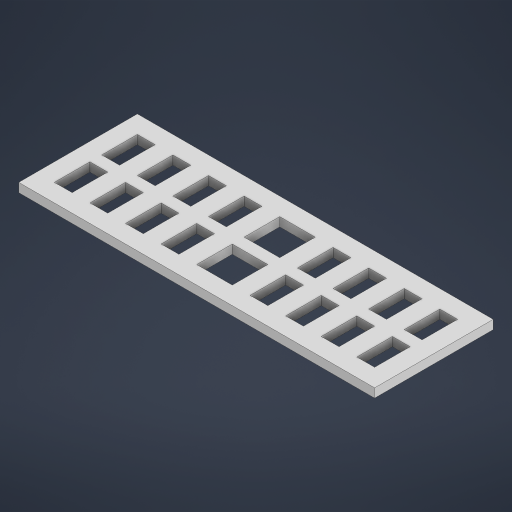
# Autodesk Inventor part: JARING
Saved by Autodesk Inventor 2024 (Build 280153000, 153)
## iProperties
Created: 2025-06-23
Part Number: JARING
Material: Generic
Document SubType Name: Modeling
Designer: ASUS
Density: 1 g/cm^3
Appearance: Default
Author: ASUS
Autodesk Inventor part; units mm, degrees
ref_plane "YZ Plane" through (0, 0, 0) normal (1, 0, 0) x (0, 1, 0)
ref_plane "XZ Plane" through (0, 0, 0) normal (0, 1, 0) x (-1, 0, 0)
ref_plane "XY Plane" through (0, 0, 0) normal (0, 0, 1) x (1, 0, 0)
sketch "Sketch1" plane through (0, 0, 0) normal (0, 1, 0) x (-1, 0, 0)
  line L0 (30, -10) -> (-30, -10)
  line L1 (-30, -10) -> (-30, 10)
  line L2 (-30, 10) -> (30, 10)
  line L3 (30, 10) -> (30, -10)
  line L4 (24, -7) -> (27, -7)
  line L5 (27, -1) -> (24, -1)
  line L6 (27, 1) -> (24, 1)
  line L7 (27, 7) -> (24, 7)
  line L8 (27, -7) -> (27, -1)
  line L9 (27, 1) -> (27, 7)
  line L10 (24, -7) -> (24, -1)
  line L11 (24, 1) -> (24, 7)
  line L12 (-27, -7) -> (-24, -7)
  line L13 (-24, -1) -> (-27, -1)
  line L14 (-24, 1) -> (-27, 1)
  line L15 (-24, 7) -> (-27, 7)
  line L16 (18, -7) -> (21, -7)
  line L17 (21, -1) -> (18, -1)
  line L18 (21, 1) -> (18, 1)
  line L19 (21, 7) -> (18, 7)
  line L20 (-21, -7) -> (-18, -7)
  line L21 (-18, -1) -> (-21, -1)
  line L22 (-18, 1) -> (-21, 1)
  line L23 (-18, 7) -> (-21, 7)
  line L24 (12, -7) -> (15, -7)
  line L25 (15, -1) -> (12, -1)
  line L26 (15, 1) -> (12, 1)
  line L27 (15, 7) -> (12, 7)
  line L28 (-15, -7) -> (-12, -7)
  line L29 (-12, -1) -> (-15, -1)
  line L30 (-12, 1) -> (-15, 1)
  line L31 (-12, 7) -> (-15, 7)
  line L32 (6, -7) -> (9, -7)
  line L33 (9, -1) -> (6, -1)
  line L34 (9, 1) -> (6, 1)
  line L35 (9, 7) -> (6, 7)
  line L36 (-9, -7) -> (-6, -7)
  line L37 (-3, -7) -> (3, -7)
  line L38 (3, -1) -> (-3, -1)
  line L39 (-6, -1) -> (-9, -1)
  line L40 (3, 1) -> (-3, 1)
  line L41 (-6, 1) -> (-9, 1)
  line L42 (3, 7) -> (-3, 7)
  line L43 (-6, 7) -> (-9, 7)
  line L44 (21, -7) -> (21, -1)
  line L45 (21, 1) -> (21, 7)
  line L46 (18, -7) -> (18, -1)
  line L47 (18, 1) -> (18, 7)
  line L48 (15, -7) -> (15, -1)
  line L49 (15, 1) -> (15, 7)
  line L50 (12, -7) -> (12, -1)
  line L51 (12, 1) -> (12, 7)
  line L52 (9, -7) -> (9, -1)
  line L53 (9, 1) -> (9, 7)
  line L54 (6, -7) -> (6, -1)
  line L55 (6, 1) -> (6, 7)
  line L56 (3, -7) -> (3, -1)
  line L57 (3, 1) -> (3, 7)
  line L58 (-3, -7) -> (-3, -1)
  line L59 (-3, 1) -> (-3, 7)
  line L60 (-6, -7) -> (-6, -1)
  line L61 (-6, 1) -> (-6, 7)
  line L62 (-9, -7) -> (-9, -1)
  line L63 (-9, 1) -> (-9, 7)
  line L64 (-12, -7) -> (-12, -1)
  line L65 (-12, 1) -> (-12, 7)
  line L66 (-15, -7) -> (-15, -1)
  line L67 (-15, 1) -> (-15, 7)
  line L68 (-18, -7) -> (-18, -1)
  line L69 (-18, 1) -> (-18, 7)
  line L70 (-21, -7) -> (-21, -1)
  line L71 (-21, 1) -> (-21, 7)
  line L72 (-24, -7) -> (-24, -1)
  line L73 (-24, 1) -> (-24, 7)
  line L74 (-27, 7) -> (-27, 1)
  line L75 (-27, -1) -> (-27, -7)
  line L76 (-27, -7) -> (-27, -1)
  line L77 (-27, 1) -> (-27, 7)
  point P0 (0, 0)
  point P1 (3, -10)
  point P2 (3, 10)
  point P3 (6, -10)
  point P4 (6, 10)
  point P5 (9, -10)
  point P6 (9, 10)
  point P7 (12, -10)
  point P8 (12, 10)
  point P9 (15, -10)
  point P10 (15, 10)
  point P11 (18, -10)
  point P12 (18, 10)
  point P13 (21, -10)
  point P14 (21, 10)
  point P15 (24, -10)
  point P16 (24, 10)
  point P17 (27, -10)
  point P18 (27, 10)
  point P19 (-3, -10)
  point P20 (-3, 10)
  point P21 (-6, -10)
  point P22 (-6, 10)
  point P23 (-9, -10)
  point P24 (-9, 10)
  point P25 (-12, -10)
  point P26 (-12, 10)
  point P27 (-15, -10)
  point P28 (-15, 10)
  point P29 (-18, -10)
  point P30 (-18, 10)
  point P31 (-21, -10)
  point P32 (-21, 10)
  point P33 (-24, -10)
  point P34 (-24, 10)
  point P35 (-27, -10)
  point P36 (-27, 10)
  constraints: 156 end point, 115 parallel, 19 perpendicular, 1 horizontal
extrude "Extrusion1" add sketch "Sketch1" along normal blind 1.5
body "Solid1"
